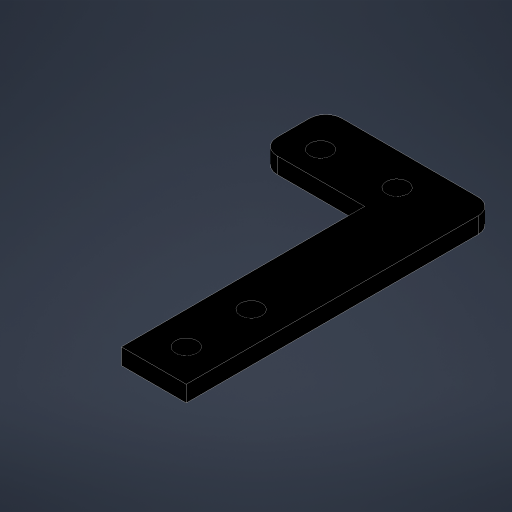
# Autodesk Inventor part: wing mount with stopper
Saved by Autodesk Inventor 2024 (Build 280153000, 153)
## iProperties
Created: 2024-01-23
Part Number: wing mount with stopper
Material: Aluminum 6061
Document SubType Name: Modeling
Designer: elite
Density: 2.7 g/cm^3
Appearance: Anodized - Black
Author: elite
Autodesk Inventor part; units mm, degrees
ref_plane "YZ Plane" through (0, 0, 0) normal (1, 0, 0) x (0, 1, 0)
ref_plane "XZ Plane" through (0, 0, 0) normal (0, 1, 0) x (-1, 0, 0)
ref_plane "XY Plane" through (0, 0, 0) normal (0, 0, 1) x (1, 0, 0)
sketch "Sketch1" plane through (0, 0, 0) normal (0, 1, 0) x (-1, 0, 0)
  line L0 (0, 0) -> (12.7, 0)
  line L1 (12.7, 0) -> (12.7, -47.625)
  line L2 (12.7, -47.625) -> (0, -47.625)
  line L3 (0, -47.625) -> (0, 0)
  line L4 (6.35, 0) -> (6.35, -6.35)
  circle A0 centre (6.35, -6.35) radius 2.1082
  line L5 (6.35, -6.35) -> (6.35, -19.05)
  circle A1 centre (6.35, -19.05) radius 2.1082
  line L6 (6.35, -19.05) -> (6.35, -53.975)
  line L7 (6.35, -53.975) -> (12.7, -53.975)
  circle A2 centre (12.7, -53.975) radius 2.1082
  line L8 (12.7, -53.975) -> (12.7, -60.325)
  line L9 (0, -47.625) -> (0, -53.975)
  line L10 (12.7, -60.325) -> (3.175, -60.325)
  line L11 (0, -57.15) -> (0, -53.975)
  arc A3 (0, -57.15) -> (3.175, -60.325) centre (3.175, -57.15) ccw
  line L12 (12.7, -53.975) -> (26.67, -53.975)
  line L13 (26.67, -53.975) -> (26.67, -52.959)
  circle A4 centre (26.67, -52.959) radius 2.1082
  line L14 (12.7, -47.625) -> (26.67, -47.625)
  line L15 (12.7, -60.325) -> (26.67, -60.325)
  line L16 (26.67, -47.625) -> (29.845, -47.625)
  line L17 (33.02, -50.8) -> (33.02, -57.15)
  line L18 (29.845, -60.325) -> (26.67, -60.325)
  arc A5 (29.845, -60.325) -> (33.02, -57.15) centre (29.845, -57.15) ccw
  arc A6 (33.02, -50.8) -> (29.845, -47.625) centre (29.845, -50.8) ccw
  point P0 (33.02, -47.625)
  dimension "d0" = 12.7
  dimension "d1" = 6.35
  dimension "d2" = 4.2164
  dimension "d3" = 47.625
  dimension "d4" = 12.7
  dimension "d5" = 34.925
  dimension "d6" = 6.35
  dimension "d7" = 4.2164
  dimension "d8" = 6.35
  dimension "d9" = 3.175
  dimension "d12" = 13.97
  dimension "d13" = 1.016
  dimension "d14" = 4.2164
  dimension "d15" = 6.35
  dimension "d16" = 3.175
  constraints: 38 end point, 7 centre point, 7 horizontal, 6 point on circle, 6 tangent, 5 perpendicular, 5 vertical, 4 coincident, 2 parallel, 2 point on line, 1 equal radius, 1 midpoint
  measures "d0" distance of L0.start L0.end
  measures "d1" distance of L4.start L4.end
  measures "d2" diameter of A0
  measures "d3" distance of L0.end L1.end
  measures "d4" distance of L5.start L5.end
  measures "d5" distance of L6.start L6.end
  measures "d6" distance of L6.end L7.end
  measures "d7" diameter of A2
  measures "d8" distance of L8.start L8.end
  measures "d9" radius of A3
  measures "d12" distance of L8.start L12.end
  measures "d13" distance of L12.end L13.end
  measures "d14" diameter of A4
  measures "d15" distance of L14.end point (33.02, -47.625)
  measures "d16" radius of A5
extrude "Extrusion1" add sketch "Sketch1" along normal blind 3.175 contours L0 L4 A0 L5 A1 L6 L2 L3 | L0 L1 L2 L6 A1 L5 A0 L4 | L2 L6 L7 A2 L8 L10 A3 L11 L9 | L2 L14 L16 A6 L17 A5 L18 L15 L8 A2 L7 L6
body "Solid1"
